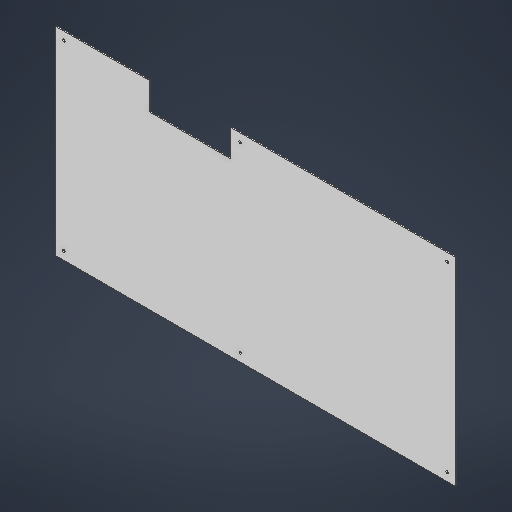
# Autodesk Inventor part: PlaqueLargeur
Saved by Autodesk Inventor 2026.2 (Build 302298010, 298A)
## iProperties
Created: 2026-05-13
Part Number: PlaqueLargeur
Material: Générique
Document SubType Name: Modeling
Designer: romai
Density: 1 g/cm^3
Appearance: Par défaut
Author: romai
Autodesk Inventor part; units mm, degrees
ref_plane "YZ Plane" through (0, 0, 0) normal (1, 0, 0) x (0, 1, 0)
ref_plane "XZ Plane" through (0, 0, 0) normal (0, 1, 0) x (-1, 0, 0)
ref_plane "XY Plane" through (0, 0, 0) normal (0, 0, 1) x (1, 0, 0)
sketch "Esquisse1" plane through (0, 0, 0) normal (0, 0, 1) x (1, 0, 0)
  line L0 (-366.5, -212.5) -> (368.5, -212.5)
  line L1 (368.5, -212.5) -> (368.5, 152.5)
  line L2 (368.5, 152.5) -> (-366.5, 152.5)
  line L3 (-366.5, 152.5) -> (-366.5, -212.5)
  line L4 (-366.5, -212.5) -> (368.5, 152.5) construction
  line L5 (-354, -200) -> (356, -200)
  line L6 (356, -200) -> (356, 140)
  line L7 (356, 140) -> (-354, 140)
  line L8 (-354, 140) -> (-354, -200)
  line L9 (-354, -200) -> (356, 140) construction
  circle A0 centre (-351.5, 137.5) radius 2.5
  circle A1 centre (-351.5, -197.5) radius 2.5
  circle A2 centre (353.5, -197.5) radius 2.5
  circle A3 centre (353.5, 137.5) radius 2.5
  point P0 (-354, -197.5)
  point P1 (-351.5, -200)
  point P2 (353.5, -200)
  point P3 (356, -197.5)
  point P4 (356, 137.5)
  point P5 (353.5, 140)
  point P6 (-354, 137.5)
  point P7 (-351.5, 140)
  dimension "d0" = 735
  dimension "d1" = 365
  dimension "d2" = 12.5
  dimension "d3" = 12.5
  dimension "d4" = 5
  dimension "d7" = 5
  dimension "d8" = 5
  dimension "d9" = 5
  dimension "d75" = 12.5
  dimension "d76" = 12.5
  constraints: 20 end point, 8 tangent, 4 centre point, 4 parallel, 2 horizontal, 2 perpendicular
  measures "d0" distance of L2.end L1.end
  measures "d1" distance of L1.end L0.end
  measures "d2" distance between parallel lines of L2 L7
  measures "d3" distance between parallel lines of L1 L6
  measures "d4" diameter of A0
  measures "d7" diameter of A1
  measures "d8" diameter of A2
  measures "d9" diameter of A3
  measures "d75" distance between parallel lines of L3 L8
  measures "d76" distance between parallel lines of L0 L5
extrude "Extrusion1" add sketch "Esquisse1" along normal blind 2 contours L3 L2 L1 L0 | L8 A1 L5 | A1 L8 A0 L7 A3 L6 A2 L5 | A2 L6 L5 | L8 L7 A0 | A3 L7 L6
sketch "Esquisse3" plane through (0, 0, 2) normal (0, 0, 1) x (1, 0, 0)
  line L0 (-194, 155.1637) -> (-44, 155.1637)
  line L1 (-44, 155.1637) -> (-44, 102.5)
  line L2 (-44, 102.5) -> (-194, 102.5)
  line L3 (-194, 102.5) -> (-194, 155.1637)
  line L4 (368.5, -212.5) -> (368.5, 152.5) projected
  line L5 (368.5, 152.5) -> (-366.5, 152.5) projected
  point P0 (0, 0)
  point P1 (-44, 128.8319)
  dimension "d65" = 412.5
  dimension "d66" = 150
  dimension "d67" = 50
  constraints: 8 end point, 2 parallel, 1 horizontal, 1 midpoint, 1 perpendicular
  measures "d65" distance from line of L4 point (-44, 128.832)
  measures "d66" distance of L1.end L2.end
  measures "d67" distance between parallel lines of L5 L2
extrude "Extrusion2" cut sketch "Esquisse3" against normal through all
sketch "Esquisse4" plane through (0, 0, 2) normal (0, 0, 1) x (1, 0, 0)
  circle A0 centre (-27, 137.5) radius 2.5
  circle A1 centre (-27, -197.5) radius 2.5
  line L0 (-29.5, 269.4833) -> (-29.5, -384.936)
  line L1 (368.5, -212.5) -> (368.5, 152.5) projected
  circle A2 centre (-351.5, -197.5) radius 2.5 projected
  circle A3 centre (-351.5, 137.5) radius 2.5 projected
  point P0 (0, 0)
  dimension "d68" = 5
  dimension "d69" = 5
  dimension "d70" = 398
  dimension "d71" = 0
  dimension "d72" = 0
  constraints: 2 centre point, 2 end point, 2 tangent, 1 vertical
  measures "d68" diameter of A0
  measures "d69" diameter of A1
  measures "d70" distance between parallel lines of L1 L0
  measures "d71" vertical distance of A2.centre A1.centre
  measures "d72" vertical distance of A3.centre A0.centre
extrude "Extrusion3" cut sketch "Esquisse4" along normal through all both and the other way through all contours A0 | A1
